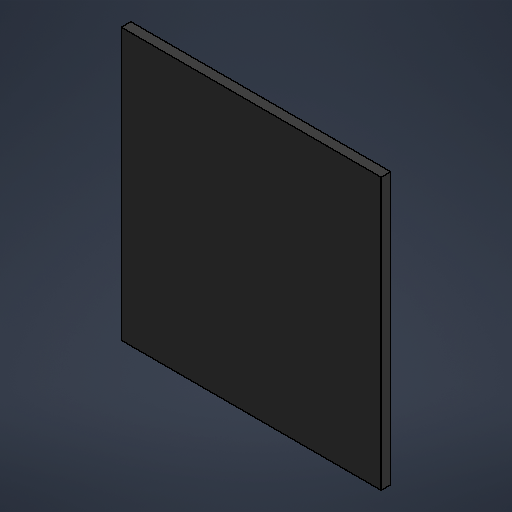
# Autodesk Inventor part: Part1
Saved by Autodesk Inventor 2026 (Build 300175050, 175E)
## iProperties
Created: 2025-05-21
Part Number: Part1
Material: Rubber
Document SubType Name: Modeling
Designer: Joshua Eah
Density: 0.93 g/cm^3
Appearance: Rubber - Black
Author: Joshua Eah
Autodesk Inventor part; units mm, degrees
ref_plane "YZ Plane" through (0, 0, 0) normal (1, 0, 0) x (0, 1, 0)
ref_plane "XZ Plane" through (0, 0, 0) normal (0, 1, 0) x (-1, 0, 0)
ref_plane "XY Plane" through (0, 0, 0) normal (0, 0, 1) x (1, 0, 0)
sketch "Sketch1" plane through (0, 0, 0) normal (0, 0, 1) x (1, 0, 0)
  line L0 (0, 0) -> (163, 0)
  line L1 (163, 0) -> (163, 170)
  line L2 (163, 170) -> (0, 170)
  line L3 (0, 170) -> (0, 0)
  dimension "d0" = 170
  dimension "d1" = 163
  constraints: 8 end point, 2 parallel, 1 horizontal, 1 perpendicular
  measures "d0" distance of L1.end L0.end
  measures "d1" distance of L0.start L0.end
extrude "Extrusion1" add sketch "Sketch1" along normal blind 6
body "Solid1"
